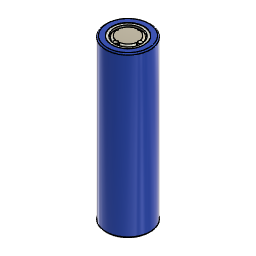
18650 (Autodesk Fusion 360 design; units mm, degrees)
Autodesk Fusion 360 part; units mm, degrees
sketch "Sketch1" plane through (0, 0, 0) normal (0, 0, 1) x (1, 0, 0)
  circle A0 centre (0, 0) radius 9
  dimension "d1" = 18
  constraint coincident A0.centre origin
  measures "d1" diameter of A0
extrude "Extrude1" add sketch "Sketch1" along normal blind 65
fillet "Fillet1" radius 0.5 2 edges at (-8.3909, -3.2545, 65) (-8.3909, -3.2545, 0)
sketch "Sketch2" plane through (0, 0, 0) normal (0, 0, -1) x (1, 0, 0)
  circle A0 centre (0, 0) radius 8.5
  circle A1 centre (0, 0) radius 5.5
  dimension "d6" = 11
  constraint concentric A0 A1
  measures "d6" diameter of A1
extrude "Extrude2" cut sketch "Sketch2" against normal blind 0.3 contours A1
sketch "Sketch3" plane through (0, 0, 65) normal (0, 0, 1) x (-1, 0, 0)
  circle A0 centre (0, 0) radius 8.5
  circle A1 centre (0, 0) radius 5.5
  circle A2 centre (0, 0) radius 6.5
  dimension "d9" = 11
  dimension "d10" = 13
  constraint coincident A0.centre A1.centre
  measures "d9" diameter of A1
  measures "d10" diameter of A2
extrude "Extrude3" cut sketch "Sketch3" against normal blind 1 contours A1
extrude "Extrude4" cut sketch "Sketch3" against normal blind 0.15 contours A2
sketch "Sketch4" plane through (0, 0, 64) normal (0, 0, 1) x (-1, 0, 0)
  circle A0 centre (0, 0) radius 5.5
  circle A1 centre (0, 0) radius 5
  dimension "d15" = 10
  constraint coincident A0.centre A1.centre
  measures "d15" diameter of A1
extrude "Extrude5" add sketch "Sketch4" along normal blind 1 contours A1
sketch "Sketch5" plane through (0, 0, 65) normal (0, 0, 1) x (-1, 0, 0)
  circle A0 centre (0, 0) radius 5
  circle A1 centre (0, 0) radius 4
  circle A2 centre (0.0101, -5.5) radius 1.5
  point P0 (0, -4)
  dimension "d18" = 8
  dimension "d19" = 3
  dimension "d26" = 5.5
  constraint concentric A0 A1
  constraint coincident A1 P0
  constraint coincident A2 P0
  measures "d18" diameter of A1
  measures "d19" diameter of A2
  measures "d26" vertical distance of A0.centre A2.centre
extrude "Extrude6" cut sketch "Sketch5" against normal blind 1 contours A0 A2 picked at (0.369, -4.6695)
pattern_circular "C-Pattern1" count 4 over 360 about axis through (0, 0, 64) along (0, 0, -1) of "Extrude6"
fillet "Fillet2" radius 0.75 4 edges at (-3.529, -3.5421, 65) (-3.5421, 3.529, 65) (3.529, 3.5421, 65) (3.5421, -3.529, 65)
named bodies: "18650"
